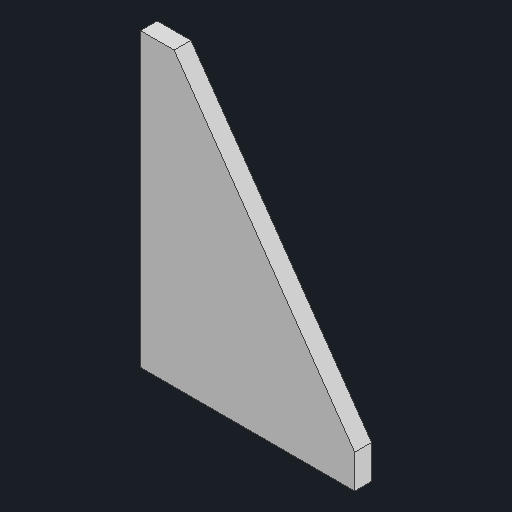
# Autodesk Inventor part: case2
Saved by Autodesk Inventor 2026.2 (Build 302298000, 298)
## iProperties
Created: 2026-01-27
Part Number: case2
Material: Generic
Document SubType Name: Modeling
Designer: mi
Density: 1 g/cm^3
Appearance: Default
Author: mi
Autodesk Inventor part; units mm, degrees
ref_plane "YZ Plane" through (0, 0, 0) normal (1, 0, 0) x (0, 1, 0)
ref_plane "XZ Plane" through (0, 0, 0) normal (0, 1, 0) x (-1, 0, 0)
ref_plane "XY Plane" through (0, 0, 0) normal (0, 0, 1) x (1, 0, 0)
sketch "Sketch1" plane through (0, 0, 0) normal (0, 0, 1) x (1, 0, 0)
  line L0 (0, 0) -> (0, 173.1814)
  line L1 (0, 173.1814) -> (20, 173.1814)
  line L2 (20, 173.1814) -> (127.2588, 20)
  line L3 (127.2588, 20) -> (127.2588, 0)
  line L4 (127.2588, 0) -> (0, 0)
  dimension "d0" = 20
  dimension "d1" = 55
  dimension "d2" = 187
  dimension "d3" = 20
  constraints: 10 end point, 2 perpendicular, 1 parallel, 1 vertical
  measures "d0" distance of L2.end L3.end
  measures "d1" angle of L4 L2
  measures "d2" distance of L1.end L2.end
  measures "d3" distance of L0.end L1.end
extrude "Extrusion1" add sketch "Sketch1" along normal blind 10
body "Solid1"
